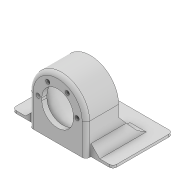
# Autodesk Inventor part: 12v DC motor mount v2
Saved by Autodesk Inventor 2022 (Build 260153000, 153)
## iProperties
Created: 2024-07-20
Part Number: 12v DC motor mount v2
Material: Generic
Document SubType Name: Modeling
Designer: david
Density: 1 g/cm^3
Appearance: Default
Author: david
Autodesk Inventor part; units mm, degrees
ref_plane "YZ Plane" through (0, 0, 0) normal (1, 0, 0) x (0, 1, 0)
ref_plane "XZ Plane" through (0, 0, 0) normal (0, 1, 0) x (-1, 0, 0)
ref_plane "XY Plane" through (0, 0, 0) normal (0, 0, 1) x (1, 0, 0)
sketch "Sketch1" plane through (0, 0, 0) normal (0, 1, 0) x (-1, 0, 0)
  line L0 (-40, 0) -> (40, 0)
  line L1 (40, 0) -> (40, -47.5)
  line L2 (40, -47.5) -> (-40, -47.5)
  line L3 (-40, -47.5) -> (-40, 0)
  line L4 (-40, 0) -> (40, -47.5) construction
  line L5 (40, 0) -> (-40, -47.5) construction
  line L6 (-56, 0) -> (56, 0) projected
  point P0 (0, 0)
  point P1 (0, -23.75)
  point P2 (0, 0)
  dimension "d0" = 47.5
  dimension "d1" = 80
  constraints: 12 end point, 3 midpoint, 2 parallel, 1 coincident, 1 collinear, 1 horizontal, 1 perpendicular
  measures "d0" distance of L2.end L0.start
  measures "d1" distance of L1.end L2.end
extrude "Extrusion1" add sketch "Sketch1" along normal blind 2
sketch "Sketch2" plane through (-40, 0, 0) normal (0, 0, 1) x (1, 0, 0)
  line L0 (40, 25) -> (40, 0) construction
  line L1 (17.5, 25) -> (17.5, 0)
  line L2 (62.5, 0) -> (62.5, 25)
  arc A0 (62.5, 25) -> (17.5, 25) centre (40, 25) ccw
  arc A1 (17.5, 0) -> (62.5, 0) centre (40, 0) ccw construction
  line L3 (0, 0) -> (80, 0) projected
  line L4 (40, 25) -> (40, 23) construction
  line L5 (27.5, 25) -> (27.5, 23)
  line L6 (52.5, 23) -> (52.5, 25)
  arc A2 (52.5, 25) -> (27.5, 25) centre (40, 25) ccw
  arc A3 (27.5, 23) -> (52.5, 23) centre (40, 23) ccw
  circle A4 centre (40, 25) radius 18.5 construction
  point P0 (40, 12.5)
  point P1 (40, 24)
  dimension "d5" = 22.5
  dimension "d6" = 2
  dimension "d7" = 25
  dimension "d27" = 37
  dimension "d28" = 6.5
  constraints: 16 end point, 8 point on circle, 8 tangent, 5 centre point, 4 midpoint, 2 coincident, 2 parallel, 1 point on line, 1 vertical
  measures "d5" radius of A0
  measures "d6" distance of L0.start L4.end
  measures "d7" diameter of A3
  measures "d27" diameter of A4
  measures "d28" distance edge to line of A4 L3
extrude "Extrusion2" add sketch "Sketch2" along normal blind 4
sketch "Sketch3" plane through (-40, 0, 0) normal (0, 0, -1) x (-1, 0, 0)
  arc A0 (-27.5, 25) -> (-52.5, 25) centre (-40, 25) ccw projected
  circle A1 centre (-40, 25) radius 19
  arc A2 (-17.5, 25) -> (-62.5, 25) centre (-40, 25) ccw projected
  line L0 (-62.5, 2) -> (-62.5, 25) projected
  line L1 (-17.5, 25) -> (-17.5, 2) projected
  line L2 (-80, 2) -> (0, 2) projected
  point P0 (-40, 0)
  dimension "d11" = 38
  constraints: 1 centre point, 1 coincident
  measures "d11" diameter of A1
extrude "Extrusion3" add sketch "Sketch3" along normal blind 22
sketch "Sketch4" plane through (-40, 0, 4) normal (0, 0, 1) x (1, 0, 0)
  circle A0 centre (40, 25) radius 15.5 construction
  arc A1 (52.5, 25) -> (27.5, 25) centre (40, 25) ccw construction
  point P0 (40, 0)
  point P1 (55.5, 25)
  point P2 (47.75, 38.4234)
  point P3 (32.25, 38.4234)
  point P4 (24.5, 25)
  point P5 (32.25, 11.5766)
  point P6 (47.75, 11.5766)
  dimension "d14" = 31
  dimension "d17" = 360
  constraints: 2 horizontal alignment, 10 other
hole "Hole1" at (15.5, 25, 4) at (7.75, 38.4234, 4) at (-15.5, 25, 4) at (-7.75, 38.4234, 4) direction (0, 0, -1) diameter 3.4 end through all
sketch "Sketch5" plane through (22.5, 0, 0) normal (1, 0, 0) x (0, 0, -1)
  line L0 (22, 2) -> (22, 25) projected
  line L1 (22, 16) -> (34, 2)
  line L2 (0, 2) -> (47.5, 2) projected
  point P0 (0, 0)
  dimension "d29" = 14
  dimension "d30" = 12
  constraints: 2 end point, 2 point on line, 1 coincident
  measures "d29" distance from line of L2 L1.start
  measures "d30" distance from line of point (34, 2) L0
extrude "Extrusion4" add sketch "Sketch5" against normal blind 3
mirror "Mirror1" about plane through (0, 0, 0) normal (1, 0, 0) of "Extrusion4"
chamfer "Chamfer1" distance 0.5 angle 45 1 edges at (19, 25, -22)
chamfer "Chamfer2" distance 3 angle 45 5 edges at (0, 2, -22) (19.5, 2, -28) (21, 2, -34) (-19.5, 2, -28) (-21, 2, -34)
chamfer "Chamfer3" distance 7 angle 45 4 edges at (22.5, 2, -35.5) (22.5, 2, -17) (-22.5, 2, -35.5) (-22.5, 2, -17)
fillet "Fillet1" radius 3 3 edges at (-22.5, 12.5, 4) (22.5, 12.5, 4) (0, 47.5, 4)
fillet "Fillet2" radius 3 5 edges at (-22.5, 4.5, 0) (-40, 1, 0) (-40, 1, -47.5) (40, 1, 0) (40, 1, -47.5)
body "Solid1"
